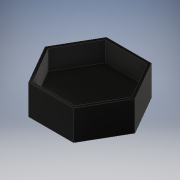
# Autodesk Inventor part: Internal Base
Saved by Autodesk Inventor 2019 (Build 230136000, 136)
## iProperties
Created: 2020-01-19
Part Number: Internal Base
Material: ABS Plastic
Document SubType Name: Modeling
Designer: prana
Density: 1.06 g/cm^3
Appearance: Smooth - White
Author: prana
Autodesk Inventor part; units mm, degrees
ref_plane "YZ Plane" through (0, 0, 0) normal (1, 0, 0) x (0, 1, 0)
ref_plane "XZ Plane" through (0, 0, 0) normal (0, 1, 0) x (-1, 0, 0)
ref_plane "XY Plane" through (0, 0, 0) normal (0, 0, 1) x (1, 0, 0)
sketch "Sketch1" plane through (0, 0, 0) normal (0, 1, 0) x (-1, 0, 0)
  line L0 (57.15, 0) -> (28.575, 49.4934)
  line L1 (28.575, 49.4934) -> (-28.575, 49.4934)
  line L2 (-28.575, 49.4934) -> (-57.15, 0)
  line L3 (57.15, 0) -> (28.575, -49.4934)
  line L4 (28.575, -49.4934) -> (-28.575, -49.4934)
  line L5 (-28.575, -49.4934) -> (-57.15, 0)
  point P0 (0, 0)
  dimension "d0" = 57.15
  dimension "d1" = 57.15
  dimension "d2" = 57.15
  dimension "d3" = 57.15
  constraints: 12 end point
  measures "d0" distance of point (0, 0) L0.start
  measures "d1" distance of L0.start L0.end
  measures "d2" distance of L0.end L1.end
  measures "d3" distance of L1.end L2.end
extrude "Extrusion1" add sketch "Sketch1" along normal blind 38.1
sketch "Sketch2" plane through (0, 38.1, 0) normal (0, 1, 0) x (1, 0, 0)
  line L0 (0, 0) -> (-53.34, 0)
  line L1 (-53.34, 0) -> (-26.67, -46.1938)
  line L2 (-26.67, -46.1938) -> (26.67, -46.1938)
  line L3 (26.67, -46.1938) -> (53.34, 0)
  line L4 (53.34, 0) -> (26.67, 46.1938)
  line L5 (26.67, 46.1938) -> (-26.67, 46.1938)
  line L6 (-26.67, 46.1938) -> (-53.34, 0)
  dimension "d6" = 53.34
  dimension "d7" = 53.34
  dimension "d8" = 60
  dimension "d9" = 53.34
  dimension "d10" = 53.34
  constraints: 14 end point, 4 parallel, 1 horizontal, 1 point on line
  measures "d6" distance of L0.start L0.end
  measures "d7" distance of L0.end L1.end
  measures "d8" angle of L1 L0
  measures "d9" distance of L1.end L2.end
  measures "d10" distance of L2.end L3.end
extrude "Extrusion2" cut sketch "Sketch2" against normal blind 31.75
sketch "Sketch3" plane through (0, 6.35, 0) normal (0, 1, 0) x (1, 0, 0)
  line L0 (26.67, -46.1938) -> (-26.67, -46.1938) projected
  line L1 (-26.67, -46.1938) -> (26.67, -46.1938)
  line L2 (53.34, 0) -> (26.67, -46.1938) projected
  line L3 (26.67, -46.1938) -> (53.34, 0)
  line L4 (-26.67, 46.1938) -> (26.67, 46.1938) projected
  line L5 (53.34, 0) -> (26.67, 46.1938)
  line L6 (26.67, 46.1938) -> (-26.67, 46.1938)
  line L7 (-26.67, 46.1938) -> (-53.34, 0)
  line L8 (-26.67, -46.1938) -> (-53.34, 0) projected
  line L9 (-53.34, 0) -> (-26.67, -46.1938)
  line L10 (-26.67, -46.1938) -> (26.67, -46.1938)
  point P0 (0, 0)
  constraints: 14 end point, 4 equal length, 1 horizontal
extrude "Extrusion3" add sketch "Sketch3" along normal blind 6.35
body "Solid1"
